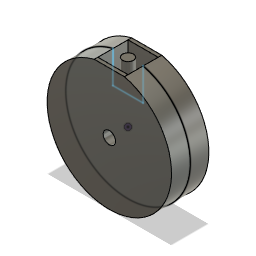
DropperContainer (Autodesk Fusion 360 design; units mm, degrees)
Autodesk Fusion 360 part; units mm, degrees
sketch "Sketch1" plane through (0, 0, 0) normal (0, 0, 1) x (1, 0, 0)
  line L0 (2.425, 4.5515) -> (-2.425, 4.5515)
  line L1 (-2.425, 4.5515) -> (-2.425, 9.7015)
  line L2 (2.425, 9.7015) -> (2.425, 4.5515)
  arc A0 (-2.425, 9.7015) -> (2.425, 9.7015) centre (0, 0) ccw
  dimension "d8" = 20
  dimension "d11" = 5.15
  dimension "d12" = 4.85
  constraint coincident A0.centre origin
  constraint perpendicular L0 L2
  measures "d8" diameter of A0
  measures "d11" distance of L2.start L0.start
  measures "d12" distance of L0.start L0.end
extrude "Extrude2" add sketch "Sketch1" along normal blind 2.5
sketch "Sketch2" plane through (0, 0, 2.5) normal (0, 0, 1) x (1, 0, 0)
  arc A0 (-2.425, 9.7015) -> (2.425, 9.7015) centre (0, 0) ccw
  line L0 (2.425, 9.7015) -> (2.425, 4.5515)
  line L1 (2.425, 4.5515) -> (-2.425, 4.5515)
  line L2 (-2.425, 4.5515) -> (-2.425, 9.7015)
  line L3 (-2.425, 9.7015) -> (2.425, 9.7015)
  line L4 (2.425, 9.7015) -> (2.425, 4.5515)
  line L5 (2.425, 4.5515) -> (-2.425, 4.5515)
  line L6 (-2.425, 4.5515) -> (-2.425, 9.7015)
  constraint horizontal L3
  constraint vertical L4
  constraint horizontal L5
  constraint vertical L6
  constraint coincident L0.end L1.start
  constraint coincident A0.start L2.end
extrude "Extrude3" add sketch "Sketch2" against normal blind 0.075 contours L0 L1 L2 L3 L4 L5 L6
extrude "Extrude4" add 1 faces at (2.4157, 4.0716, 2.5) along direction (0, 0, 1) blind 0.5
mirror "Mirror1" about plane through (0, 0, 0) normal (0, 0, -1) of bodies 1 merged
sketch "Sketch5" plane through (0, 4.5515, 0) normal (0, 1, 0) x (-1, 0, 0)
  line L0 (2.425, 2.425) -> (-2.425, 2.425)
  line L1 (-2.425, 2.425) -> (-2.425, -2.425)
  line L2 (-2.425, -2.425) -> (2.425, -2.425)
  line L3 (2.425, -2.425) -> (2.425, 2.425)
  circle A0 centre (0, 0) radius 0.875
  dimension "d29" = 1.75
  constraint coincident A0.centre origin
  measures "d29" diameter of A0
extrude "Extrude6" add sketch "Sketch5" along normal blind 5.15 contours A0
sketch "Sketch7" plane through (0, 0, 3) normal (0, 0, 1) x (1, 0, 0)
  arc A0 (-2.425, 9.7015) -> (2.425, 9.7015) centre (0, 0) ccw
  line L0 (2.425, 9.7015) -> (-2.425, 9.7015)
  circle A1 centre (0, 0) radius 1
  dimension "d32" = 2
  constraint coincident A0.centre A1.centre
  measures "d32" diameter of A1
extrude "Extrude7" cut sketch "Sketch7" against normal blind 6 contours A1
shell "Shell4" thickness 2 removed faces 0 bodies 1
sketch "Sketch3" plane through (0, 4.5515, 0) normal (0, 1, 0) x (-1, 0, 0)
  line L0 (2.425, 2.425) -> (-2.425, 2.425)
  line L1 (-2.425, 2.425) -> (-2.425, -2.425)
  line L2 (-2.425, -2.425) -> (2.425, -2.425)
  line L3 (2.425, -2.425) -> (2.425, 2.425)
  circle A0 centre (0, 0) radius 1
  dimension "d24" = 2
  constraint coincident A0.centre origin
  measures "d24" diameter of A0
extrude "Extrude5" [suppressed]
shell "Shell3" [suppressed]
shell "Shell2" [suppressed]
fillet "Fillet1" [suppressed]
extrude "Extrude1" [suppressed]
shell "Shell1" [suppressed]
